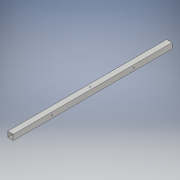
# Autodesk Inventor part: 1x1 29in
Saved by Autodesk Inventor 2018 (Build 220112000, 112)
## iProperties
Created: 2019-01-13
Part Number: 1x1 29in
Material: Generic
Document SubType Name: Modeling
Designer: s-2512711
Density: 1 g/cm^3
Appearance: Default
Author: s-2512711
Autodesk Inventor part; units mm, degrees
ref_plane "YZ Plane" through (0, 0, 0) normal (1, 0, 0) x (0, 1, 0)
ref_plane "XZ Plane" through (0, 0, 0) normal (0, 1, 0) x (-1, 0, 0)
ref_plane "XY Plane" through (0, 0, 0) normal (0, 0, 1) x (1, 0, 0)
sketch "Sketch1" plane through (0, 0, 0) normal (0, 0, 1) x (1, 0, 0)
  line L0 (0, 0) -> (25.4, 0)
  line L1 (25.4, 0) -> (25.4, 25.4)
  line L2 (25.4, 25.4) -> (0, 25.4)
  line L3 (0, 25.4) -> (0, 0)
  line L4 (3.175, 22.225) -> (22.225, 22.225)
  line L5 (22.225, 22.225) -> (22.225, 3.175)
  line L6 (22.225, 3.175) -> (3.175, 3.175)
  line L7 (3.175, 3.175) -> (3.175, 22.225)
  dimension "d0" = 25.4
  dimension "d1" = 25.4
  dimension "d2" = 3.175
  constraints: 16 end point, 4 parallel, 2 perpendicular, 1 horizontal, 3 other
  measures "d0" distance of L2.end L1.end
  measures "d1" distance of L1.end L0.end
  measures "d2" distance between parallel lines of L2 L4
extrude "Extrusion1" add sketch "Sketch1" along normal blind 736.6
sketch "Sketch2" plane through (25.4, 0, 0) normal (1, 0, 0) x (0, 0, -1)
  line L0 (0, 22.225) -> (0, 3.175) construction
  line L1 (0, 12.7) -> (-177.8, 12.7) construction
  line L2 (-736.6, 25.4) -> (-736.6, 0) construction
  line L3 (-736.6, 12.7) -> (-558.8, 12.7) construction
  circle A0 centre (-558.8, 12.7) radius 2.5797
  circle A1 centre (-177.8, 12.7) radius 2.5797
  point P0 (0, 0)
  dimension "d5" = 177.8
  dimension "d6" = 177.8
  dimension "d7" = 5.1594
  constraints: 4 end point, 2 centre point, 2 coincident, 2 horizontal, 2 midpoint
  measures "d5" distance of L1.start L1.end
  measures "d6" distance of L3.start L3.end
  measures "d7" diameter of A0
extrude "Extrusion2" cut sketch "Sketch2" against normal blind 25.4
sketch "Sketch3" plane through (0, 25.4, 0) normal (0, 1, 0) x (1, 0, 0)
  line L0 (0, 0) -> (0, -736.6) construction
  line L1 (0, -368.3) -> (25.4, -368.3) construction
  line L2 (0, -368.3) -> (25.4, -368.3) construction
  circle A0 centre (12.7, -368.3) radius 2.5797
  dimension "d10" = 25.4
  dimension "d11" = 0
  dimension "d12" = 5.1594
  constraints: 4 end point, 2 midpoint, 1 centre point, 1 collinear, 1 horizontal, 1 perpendicular
  measures "d10" distance of L1.start L1.end
  measures "d11" distance between parallel lines of L1 L2
  measures "d12" diameter of A0
extrude "Extrusion3" cut sketch "Sketch3" against normal blind 25.4
body "Solid1"
